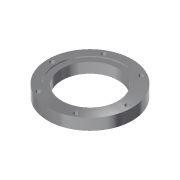
# Autodesk Inventor part: Membranring_BFA_35_30_10
Saved by Autodesk Inventor 2018.3 (Build 223284000, 284)
## iProperties
Created: 2016-11-15
Part Number: Membranring_BFA_35_30_10
Material: Stahl, Legierung
Document SubType Name: Modeling
Designer: stud_brinkmann
Density: 7.73 g/cm^3
Appearance: Halbpoliert
Mass: 28.5465 g
Surface Area: 43.6116 cm^2
Volume: 3.69295 cm^3
Author: stud_brinkmann
Autodesk Inventor part; units mm, degrees
ref_plane "YZ Plane" through (0, 0, 0) normal (1, 0, 0) x (0, 1, 0)
ref_plane "XZ Plane" through (0, 0, 0) normal (0, 1, 0) x (-1, 0, 0)
ref_plane "XY Plane" through (0, 0, 0) normal (0, 0, 1) x (1, 0, 0)
sketch "Skizze4" plane through (0, 0, 0) normal (0, 0, 1) x (1, 0, 0)
  circle A0 centre (0, 0) radius 31.5
  circle A1 centre (0, 0) radius 21
  dimension "d18" = 63
  dimension "d19" = 10.5
  constraints: 2 centre point, 2 coincident
  measures "d18" diameter of A0
  measures "d19" radial gap between concentric circles of A1 A0
extrude "Extrusion2" add sketch "Skizze4" against normal blind 8.5
sketch "Skizze9" plane through (0, 0, 0) normal (0, 0, 1) x (1, 0, 0)
  circle A0 centre (0, 0) radius 25.3
  dimension "d35" = 50.6
  constraints: 1 centre point, 1 coincident
  measures "d35" diameter of A0
extrude "Extrusion3" cut sketch "Skizze9" against normal blind 0.8
sketch "Skizze10" plane through (0, 0, -8.5) normal (0, 0, -1) x (-1, 0, 0)
  line L0 (0, 0) -> (-28.15, 0) construction
  point P0 (-14.075, -24.3786)
  point P1 (14.075, -24.3786)
  point P2 (28.15, 0)
  point P3 (14.075, 24.3786)
  point P4 (-14.075, 24.3786)
  dimension "d38" = 28.15
  dimension "d41" = 360
  constraints: 2 end point, 1 coincident, 1 horizontal, 7 other
  measures "d38" distance of L0.start L0.end
sketch "Skizze11" plane through (0, 0, -8.5) normal (0, 0, -1) x (-1, 0, 0)
  point P0 (-28.15, 0)
  point P1 (-14.075, -24.3786)
  point P2 (14.075, -24.3786)
  point P3 (14.075, 24.3786)
  point P4 (-14.075, 24.3786)
  point P5 (28.15, 0)
hole "Bohrung3" at (28.15, 0, -8.5) at (14.075, -24.3786, -8.5) at (-14.075, -24.3786, -8.5) at (-14.075, 24.3786, -8.5) at (14.075, 24.3786, -8.5) at (-28.15, 0, -8.5) direction (0, 0, 1) diameter 3.4 depth 8.5
